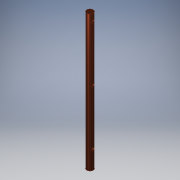
# Autodesk Inventor part: cu_stange
Saved by Autodesk Inventor 2017 (Build 210142000, 142)
## iProperties
Part Number: cu_stange
Material: Generisch
Document SubType Name: Modeling
Designer: Philomena-Theresa
Density: 1 g/cm^3
Appearance: Vorgabe
Author: Philomena-Theresa
Autodesk Inventor part; units mm, degrees
ref_plane "XZ Plane" through (0, 0, 0) normal (0, 1, 0) x (-1, 0, 0)
ref_plane "XY Plane" through (0, 0, 0) normal (0, 0, 1) x (1, 0, 0)
sketch "Skizze1" plane through (0, 0, 0) normal (0, 0, 1) x (1, 0, 0)
  circle A0 centre (0, 0) radius 1.75
  dimension "d0" = 3.5
  constraints: 1 centre point, 1 coincident
  measures "d0" diameter of A0
extrude "Extrusion1" add sketch "Skizze1" along normal blind 75
ref_plane "Arbeitsebene2" through (1.75, 0, 0) normal (1, 0, 0) x (0, 1, 0)
sketch "Skizze8" plane through (1.75, 0, 0) normal (1, 0, 0) x (0, 1, 0)
  line L0 (0, 0) -> (0, 10) construction
  line L1 (0, 10) -> (0, 40.5) construction
  line L2 (0, 40.5) -> (0, 71) construction
  dimension "d14" = 10
  dimension "d15" = 30.5
  dimension "d16" = 30.5
  constraints: 6 end point, 3 coincident, 2 point on line, 1 vertical
  measures "d14" distance of L0.start L0.end
  measures "d15" distance of L0.end L1.end
  measures "d16" distance of L1.end L2.end
hole "Bohrung2" at (1.75, 0, 10) at (1.75, 0, 40.5) at (1.75, 0, 71) at (1.75, 0, 10) at (1.75, 0, 40.5) at (1.75, 0, 71) direction (-1, 0, 0) diameter 1.6 depth 2 tip angle 118 clearance for "Flachkopfmaschinenschraube (82)" size "#0" standard "ANSI UST"
